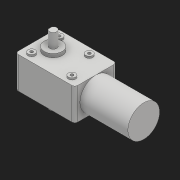
# Autodesk Inventor part: TJW83FZY4468-527i
Saved by Autodesk Inventor 2017 (Build 210142000, 142)
## iProperties
Created: 2019-09-13
Part Number: TJW83FZY4468-527i
Material: Generic
Document SubType Name: Modeling
Designer: Dell
Density: 1 g/cm^3
Appearance: Default
Author: Dell
Autodesk Inventor part; units mm, degrees
ref_plane "YZ Plane" through (0, 0, 0) normal (1, 0, 0) x (0, 1, 0)
ref_plane "XZ Plane" through (0, 0, 0) normal (0, 1, 0) x (-1, 0, 0)
ref_plane "XY Plane" through (0, 0, 0) normal (0, 0, 1) x (1, 0, 0)
sketch "Sketch1" plane through (0, 0, 0) normal (0, 0, 1) x (1, 0, 0)
  line L0 (0, 0) -> (82.5, 0)
  line L1 (82.5, 0) -> (82.5, 58)
  line L2 (82.5, 58) -> (0, 58)
  line L3 (0, 58) -> (0, 0)
  line L4 (12.6, 10) -> (68.5, 10) construction
  line L5 (68.5, 10) -> (68.5, 48) construction
  line L6 (68.5, 48) -> (12.6, 48) construction
  line L7 (12.6, 48) -> (12.6, 10) construction
  circle A0 centre (12.6, 48) radius 2
  circle A1 centre (12.6, 10) radius 2
  circle A2 centre (68.5, 10) radius 2
  circle A3 centre (54.5, 48) radius 2
  circle A4 centre (23.5, 29) radius 12.5
  circle A5 centre (23.5, 29) radius 5
  point P0 (12.6, 29)
  point P1 (0, 29)
  dimension "d0" = 82.5
  dimension "d1" = 58
  dimension "d2" = 38
  dimension "d3" = 55.9
  dimension "d4" = 12.6
  dimension "d5" = 4
  dimension "d6" = 4
  dimension "d7" = 4
  dimension "d8" = 4
  dimension "d9" = 25
  dimension "d10" = 41.9
  dimension "d11" = 10.9
  dimension "d12" = 10
  constraints: 16 end point, 6 centre point, 4 coincident, 4 parallel, 2 horizontal, 2 horizontal alignment, 2 midpoint, 2 perpendicular, 1 point on line
  measures "d0" distance of L2.end L1.end
  measures "d1" distance of L1.end L0.end
  measures "d2" distance of L6.end L4.start
  measures "d3" distance of L4.start L4.end
  measures "d4" distance between parallel lines of L3 L7
  measures "d5" diameter of A0
  measures "d6" diameter of A1
  measures "d7" diameter of A2
  measures "d8" diameter of A3
  measures "d9" diameter of A4
  measures "d10" distance of A3.centre L6.end
  measures "d11" distance from line of L7 A4.centre
  measures "d12" diameter of A5
extrude "Extrusion1" add sketch "Sketch1" along normal blind 44 contours L3 L2 L1 L0 | A4 | A5
extrude "Extrusion2" add sketch "Sketch1" along normal blind 49 and the other way blind 5 contours A4
extrude "Extrusion3" add sketch "Sketch1" against normal blind 25 and the other way blind 69 contours A5
sketch "Sketch2" plane through (0, 0, 44) normal (0, 0, 1) x (1, 0, 0)
  circle A0 centre (12.6, 48) radius 2 projected
  circle A1 centre (54.5, 48) radius 2 projected
  circle A2 centre (68.5, 10) radius 2 projected
  circle A3 centre (12.6, 10) radius 2 projected
  circle A4 centre (12.6, 48) radius 5
  circle A5 centre (54.5, 48) radius 5
  circle A6 centre (68.5, 10) radius 5
  circle A7 centre (12.6, 10) radius 5
  point P0 (0, 0)
  dimension "d23" = 10
  dimension "d24" = 10
  dimension "d25" = 10
  dimension "d26" = 10
  constraints: 4 centre point, 4 coincident
  measures "d23" diameter of A4
  measures "d24" diameter of A5
  measures "d25" diameter of A6
  measures "d26" diameter of A7
extrude "Extrusion4" add sketch "Sketch2" along normal blind 2.5
sketch "Sketch3" plane through (0, 0, 0) normal (0, 0, -1) x (-1, 0, 0)
  circle A0 centre (-12.6, 48) radius 2 projected
  circle A1 centre (-12.6, 48) radius 5 projected
  circle A2 centre (-12.6, 10) radius 2 projected
  circle A3 centre (-12.6, 10) radius 5 projected
  circle A4 centre (-54.5, 48) radius 2 projected
  circle A5 centre (-54.5, 48) radius 5 projected
  circle A6 centre (-68.5, 10) radius 2 projected
  circle A7 centre (-68.5, 10) radius 5 projected
  point P0 (0, 0)
extrude "Extrusion5" add sketch "Sketch3" along normal blind 2.5
sketch "Sketch4" plane through (82.5, 0, 0) normal (1, 0, 0) x (0, 0, -1)
  circle A0 centre (-22, 29) radius 22
  line L0 (0, 0) -> (0, 58) projected
  line L1 (0, 58) -> (-44, 58) projected
  point P0 (-22, 58)
  point P1 (0, 29)
  dimension "d31" = 44
  constraints: 2 midpoint, 1 centre point, 1 horizontal alignment, 1 vertical alignment
  measures "d31" diameter of A0
extrude "Extrusion6" add sketch "Sketch4" along normal blind 66.5
sketch "Sketch5" plane through (23.5, 29, -25) normal (0, 0, -1) x (-1, 0, 0)
  circle A0 centre (0, 0) radius 5 projected
  line L0 (4.25, -2.6339) -> (4.25, 2.6339)
  arc A1 (4.25, -2.6339) -> (4.25, 2.6339) centre (0, 0) ccw
  point P0 (23.5, -29)
  point P1 (4.25, 0)
  dimension "d34" = 4.25
  constraints: 4 point on circle, 2 end point, 1 centre point, 1 concentric, 1 horizontal alignment, 1 midpoint, 1 vertical
  measures "d34" distance from line of A0.centre L0
extrude "Extrusion7" cut sketch "Sketch5" against normal blind 15 contours A0 L0 picked at (4.3873, -0.6025)
sketch "Sketch6" plane through (23.5, 29, 69) normal (0, 0, 1) x (1, 0, 0)
  circle A0 centre (0, 0) radius 5 projected
  line L0 (-4.25, 2.6339) -> (-4.25, -2.6339)
  arc A1 (-4.25, 2.6339) -> (-4.25, -2.6339) centre (0, 0) ccw
  point P0 (-23.5, -29)
  point P1 (-4.25, 0)
  dimension "d37" = 4.25
  constraints: 4 point on circle, 2 end point, 1 centre point, 1 concentric, 1 horizontal alignment, 1 midpoint, 1 vertical
  measures "d37" distance from line of A0.centre L0
extrude "Extrusion8" cut sketch "Sketch6" against normal blind 15 contours L0 A0 picked at (-4.4085, 0.5446)
fillet "Fillet1" radius 4 4 edges at (82.5, 58, 22) (0, 58, 22) (82.5, 0, 22) (0, 0, 22)
body "Solid1"
